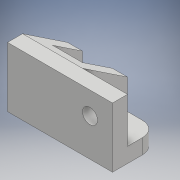
# Autodesk Inventor part: 31
Saved by Autodesk Inventor 2017 (Build 210142000, 142)
## iProperties
Part Number: 31
Material: 一般
Document SubType Name: Modeling
Designer: Brian
Density: 1 g/cm^3
Appearance: 預設
Author: Brian
Autodesk Inventor part; units mm, degrees
ref_plane "YZ Plane" through (0, 0, 0) normal (1, 0, 0) x (0, 1, 0)
ref_plane "XZ Plane" through (0, 0, 0) normal (0, 1, 0) x (-1, 0, 0)
ref_plane "XY Plane" through (0, 0, 0) normal (0, 0, 1) x (1, 0, 0)
sketch "草圖1" plane through (0, 0, 0) normal (0, 1, 0) x (-1, 0, 0)
  line L0 (0, 0) -> (-70, 0)
  line L1 (-70, 0) -> (-70, -40)
  line L2 (-70, -40) -> (0, -40)
  line L3 (0, -40) -> (0, 0)
  dimension "d0" = 40
  dimension "d1" = 70
  constraints: 8 end point, 2 parallel, 1 horizontal, 1 perpendicular
  measures "d0" distance of L2.end L0.start
  measures "d1" distance of L1.end L2.end
extrude "擠出1" add sketch "草圖1" along normal blind 10
sketch "草圖2" plane through (0, 0, 0) normal (0, 0, 1) x (1, 0, 0)
  line L0 (0, 0) -> (0, 10) projected
  line L1 (0, 10) -> (10, 10)
  line L2 (10, 10) -> (10, 40)
  line L3 (10, 40) -> (0, 40)
  line L4 (0, 40) -> (0, 10)
  line L5 (10, 10) -> (30, 10)
  line L6 (30, 10) -> (30, 20)
  line L7 (30, 20) -> (10, 20)
  line L8 (10, 20) -> (10, 10)
  line L9 (30, 10) -> (40, 10)
  line L10 (40, 10) -> (40, 40)
  line L11 (40, 40) -> (30, 40)
  line L12 (30, 40) -> (30, 10)
  dimension "d4" = 20
  dimension "d5" = 10
  dimension "d6" = 10
  dimension "d7" = 10
  dimension "d8" = 30
  constraints: 24 end point, 6 parallel, 3 horizontal, 3 perpendicular, 1 point on line
  measures "d4" distance of L6.end L7.end
  measures "d5" distance of L10.end L11.end
  measures "d6" distance of L2.end L3.end
  measures "d7" distance between parallel lines of L5 L7
  measures "d8" distance of L3.end L0.end
extrude "擠出2" add sketch "草圖2" against normal blind 40
sketch "草圖3" plane through (70, 0, -40) normal (0, 0, -1) x (-1, 0, 0)
  line L0 (30, 10) -> (30, 40) projected
  line L1 (30, 10) -> (0, 10)
  line L2 (0, 10) -> (0, 30)
  line L3 (0, 30) -> (30, 30)
  line L4 (30, 30) -> (30, 10)
  point P0 (70, 0)
  dimension "d11" = 20
  dimension "d12" = 30
  constraints: 8 end point, 2 parallel, 1 horizontal, 1 perpendicular
  measures "d11" distance of L1.end L2.end
  measures "d12" distance of L2.end L3.end
extrude "擠出3" add sketch "草圖3" against normal blind 10
fillet "圓角1" radius 10 1 edges at (70, 30, -35)
sketch "草圖4" plane through (40, 10, 0) normal (1, 0, 0) x (0, 0, -1)
  line L0 (0, 0) -> (0, 30) projected
  line L1 (0, 0) -> (20, 30)
  line L2 (20, 30) -> (0, 30)
  point P0 (0, -10)
  dimension "d16" = 20
  dimension "d17" = 30
  constraints: 4 end point
  measures "d16" horizontal distance of L0.start L1.end
  measures "d17" vertical distance of L0.start L1.end
extrude "擠出4" cut sketch "草圖4" against normal through all
sketch "草圖5" plane through (0, 10, 0) normal (0, 1, 0) x (1, 0, 0)
  circle A0 centre (55, 15) radius 5
  line L0 (70, 0) -> (70, 30) projected
  line L1 (40, 0) -> (70, 0) projected
  point P0 (0, 0)
  dimension "d20" = 15
  dimension "d21" = 15
  dimension "d22" = 10
  constraints: 1 centre point
  measures "d20" distance from line of L0 A0.centre
  measures "d21" distance from line of L1 A0.centre
  measures "d22" diameter of A0
extrude "擠出5" cut sketch "草圖5" against normal blind 10
